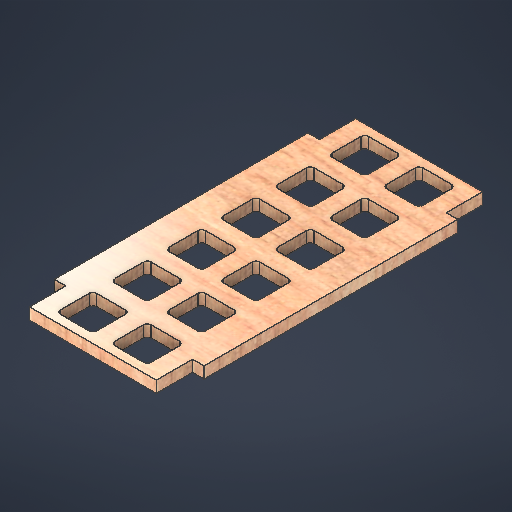
# Autodesk Inventor part: Base-Skiba
Saved by Autodesk Inventor 2027.1 (Build 311270010, 270A)
## iProperties
Created: 2025-11-09
Part Number: Base-Skiba
Material: Generic
Document SubType Name: Modeling
Designer: Nick
Density: 1 g/cm^3
Appearance: Birch - Natural Polished
Mass: 61.0819 g
Surface Area: 284.091 cm^2
Volume: 61.0819 cm^3
Author: Nick
Autodesk Inventor part; units mm, degrees
ref_plane "YZ Plane" through (0, 0, 0) normal (1, 0, 0) x (0, 1, 0)
ref_plane "XZ Plane" through (0, 0, 0) normal (0, 1, 0) x (-1, 0, 0)
ref_plane "XY Plane" through (0, 0, 0) normal (0, 0, 1) x (1, 0, 0)
sketch "Sketch1" plane through (0, 0, 0) normal (0, 1, 0) x (-1, 0, 0)
  line L0 (0, 0) -> (70, 0)
  line L1 (70, 0) -> (70, -180)
  line L2 (70, -180) -> (0, -180)
  line L3 (0, -180) -> (0, 0)
  line L4 (0, 0) -> (4.5, 0)
  line L5 (4.5, 0) -> (4.5, -10) construction
  line L6 (4.5, -10) -> (0, -10) construction
  line L7 (0, -10) -> (0, 0)
  line L8 (4.5, -10) -> (10.85, -10)
  line L9 (10.85, -10) -> (10.85, -30)
  line L10 (10.85, -30) -> (4.5, -30)
  line L11 (4.5, -30) -> (4.5, -10)
  line L12 (4.5, -80) -> (10.85, -80)
  line L13 (10.85, -80) -> (10.85, -100)
  line L14 (10.85, -100) -> (4.5, -100)
  line L15 (4.5, -100) -> (4.5, -80)
  line L16 (4.5, -150) -> (10.85, -150)
  line L17 (10.85, -150) -> (10.85, -170)
  line L18 (10.85, -170) -> (4.5, -170)
  line L19 (4.5, -170) -> (4.5, -150)
  line L20 (35, 0) -> (35, -180) construction
  line L21 (0, -20) -> (-6.35, -20)
  line L22 (-6.35, -20) -> (-6.35, -160)
  line L23 (-6.35, -160) -> (0, -160)
  line L24 (0, -160) -> (0, -20)
  line L25 (65.5, -170) -> (65.5, -150)
  line L26 (70, -20) -> (76.35, -20)
  line L27 (76.35, -20) -> (76.35, -160)
  line L28 (76.35, -160) -> (70, -160)
  line L29 (70, -160) -> (70, -20)
  point P0 (70, -160)
  dimension "d0" = 70
  dimension "d1" = 180
  dimension "d2" = 4.5
  dimension "d3" = 10
  dimension "d8" = 70
  dimension "d30" = 6.35
  dimension "d31" = 140
  constraints: 60 end point, 8 parallel, 6 symmetric about line, 4 horizontal, 4 perpendicular, 2 midpoint, 1 point on line, 1 vertical, 16 other
  measures "d0" distance of L1.end L2.end
  measures "d1" distance of L0.end L1.end
  measures "d2" distance of L5.end L6.end
  measures "d3" distance of L4.end L5.end
  measures "d8" distance of L5.end L12.start
  measures "d30" distance of L23.end L22.end
  measures "d31" distance of L22.end L21.end
extrude "Extrusion1" add sketch "Sketch1" along normal blind 6.35 contours L0 L1 L2 L3 | L3 L23 L22 L21 | L26 L27 L28 L1 | L8 L9 L10 L11 | L12 L13 L14 L15 | L16 L17 L18 L19
sketch "Sketch2" plane through (0, 6.35, 0) normal (0, 1, 0) x (1, 0, 0)
  line L0 (-70, 180) -> (-70, 0) construction
  line L1 (-70, 0) -> (-60, 0) construction
  line L2 (-60, 0) -> (-60, 5) construction
  line L3 (-60, 5) -> (-70, 5) construction
  line L4 (-70, 5) -> (-70, 0) construction
  line L5 (-58, 5) -> (-42, 5)
  line L6 (-40, 7) -> (-40, 23)
  line L7 (-42, 25) -> (-58, 25)
  line L8 (-60, 23) -> (-60, 7)
  arc A0 (-58, 25) -> (-60, 23) centre (-58, 23) ccw
  arc A1 (-42, 5) -> (-40, 7) centre (-42, 7) ccw
  arc A2 (-40, 23) -> (-42, 25) centre (-42, 23) ccw
  arc A3 (-60, 7) -> (-58, 5) centre (-58, 7) ccw
  arc A4 (-60, 37) -> (-58, 35) centre (-58, 37) ccw
  arc A5 (-42, 35) -> (-40, 37) centre (-42, 37) ccw
  line L9 (-60, 53) -> (-60, 37)
  line L10 (-42, 55) -> (-58, 55)
  arc A6 (-58, 55) -> (-60, 53) centre (-58, 53) ccw
  arc A7 (-40, 53) -> (-42, 55) centre (-42, 53) ccw
  line L11 (-40, 37) -> (-40, 53)
  line L12 (-58, 35) -> (-42, 35)
  arc A8 (-60, 67) -> (-58, 65) centre (-58, 67) ccw
  arc A9 (-42, 65) -> (-40, 67) centre (-42, 67) ccw
  line L13 (-60, 83) -> (-60, 67)
  line L14 (-42, 85) -> (-58, 85)
  arc A10 (-58, 85) -> (-60, 83) centre (-58, 83) ccw
  arc A11 (-40, 83) -> (-42, 85) centre (-42, 83) ccw
  line L15 (-40, 67) -> (-40, 83)
  line L16 (-58, 65) -> (-42, 65)
  arc A12 (-60, 97) -> (-58, 95) centre (-58, 97) ccw
  arc A13 (-42, 95) -> (-40, 97) centre (-42, 97) ccw
  line L17 (-60, 113) -> (-60, 97)
  line L18 (-42, 115) -> (-58, 115)
  arc A14 (-58, 115) -> (-60, 113) centre (-58, 113) ccw
  arc A15 (-40, 113) -> (-42, 115) centre (-42, 113) ccw
  line L19 (-40, 97) -> (-40, 113)
  line L20 (-58, 95) -> (-42, 95)
  arc A16 (-30, 7) -> (-28, 5) centre (-28, 7) ccw
  arc A17 (-12, 5) -> (-10, 7) centre (-12, 7) ccw
  line L21 (-30, 23) -> (-30, 7)
  line L22 (-12, 25) -> (-28, 25)
  arc A18 (-28, 25) -> (-30, 23) centre (-28, 23) ccw
  arc A19 (-10, 23) -> (-12, 25) centre (-12, 23) ccw
  line L23 (-10, 7) -> (-10, 23)
  line L24 (-28, 5) -> (-12, 5)
  arc A20 (-30, 37) -> (-28, 35) centre (-28, 37) ccw
  arc A21 (-12, 35) -> (-10, 37) centre (-12, 37) ccw
  line L25 (-30, 53) -> (-30, 37)
  line L26 (-12, 55) -> (-28, 55)
  arc A22 (-28, 55) -> (-30, 53) centre (-28, 53) ccw
  arc A23 (-10, 53) -> (-12, 55) centre (-12, 53) ccw
  line L27 (-10, 37) -> (-10, 53)
  line L28 (-28, 35) -> (-12, 35)
  arc A24 (-30, 67) -> (-28, 65) centre (-28, 67) ccw
  arc A25 (-12, 65) -> (-10, 67) centre (-12, 67) ccw
  line L29 (-30, 83) -> (-30, 67)
  line L30 (-12, 85) -> (-28, 85)
  arc A26 (-28, 85) -> (-30, 83) centre (-28, 83) ccw
  arc A27 (-10, 83) -> (-12, 85) centre (-12, 83) ccw
  line L31 (-10, 67) -> (-10, 83)
  line L32 (-28, 65) -> (-12, 65)
  arc A28 (-30, 97) -> (-28, 95) centre (-28, 97) ccw
  arc A29 (-12, 95) -> (-10, 97) centre (-12, 97) ccw
  line L33 (-30, 113) -> (-30, 97)
  line L34 (-12, 115) -> (-28, 115)
  arc A30 (-28, 115) -> (-30, 113) centre (-28, 113) ccw
  arc A31 (-10, 113) -> (-12, 115) centre (-12, 113) ccw
  line L35 (-10, 97) -> (-10, 113)
  line L36 (-28, 95) -> (-12, 95)
  arc A32 (-60, 127) -> (-58, 125) centre (-58, 127) ccw
  arc A33 (-42, 125) -> (-40, 127) centre (-42, 127) ccw
  line L37 (-60, 143) -> (-60, 127)
  line L38 (-42, 145) -> (-58, 145)
  arc A34 (-58, 145) -> (-60, 143) centre (-58, 143) ccw
  arc A35 (-40, 143) -> (-42, 145) centre (-42, 143) ccw
  line L39 (-40, 127) -> (-40, 143)
  line L40 (-58, 125) -> (-42, 125)
  arc A36 (-30, 127) -> (-28, 125) centre (-28, 127) ccw
  arc A37 (-12, 125) -> (-10, 127) centre (-12, 127) ccw
  line L41 (-30, 143) -> (-30, 127)
  line L42 (-12, 145) -> (-28, 145)
  arc A38 (-28, 145) -> (-30, 143) centre (-28, 143) ccw
  arc A39 (-10, 143) -> (-12, 145) centre (-12, 143) ccw
  line L43 (-10, 127) -> (-10, 143)
  line L44 (-28, 125) -> (-12, 125)
  arc A40 (-60, 157) -> (-58, 155) centre (-58, 157) ccw
  arc A41 (-42, 155) -> (-40, 157) centre (-42, 157) ccw
  line L45 (-60, 173) -> (-60, 157)
  line L46 (-42, 175) -> (-58, 175)
  arc A42 (-58, 175) -> (-60, 173) centre (-58, 173) ccw
  arc A43 (-40, 173) -> (-42, 175) centre (-42, 173) ccw
  line L47 (-40, 157) -> (-40, 173)
  line L48 (-58, 155) -> (-42, 155)
  arc A44 (-30, 157) -> (-28, 155) centre (-28, 157) ccw
  arc A45 (-12, 155) -> (-10, 157) centre (-12, 157) ccw
  line L49 (-30, 173) -> (-30, 157)
  line L50 (-12, 175) -> (-28, 175)
  arc A46 (-28, 175) -> (-30, 173) centre (-28, 173) ccw
  arc A47 (-10, 173) -> (-12, 175) centre (-12, 173) ccw
  line L51 (-10, 157) -> (-10, 173)
  line L52 (-28, 155) -> (-12, 155)
  point P0 (0, 0)
  point P1 (-40, 25)
  point P2 (-40, 5)
  point P3 (-60, 25)
  point P4 (-40, 35)
  point P5 (-60, 55)
  point P6 (-60, 35)
  point P7 (-40, 55)
  point P8 (-40, 65)
  point P9 (-60, 85)
  point P10 (-60, 65)
  point P11 (-40, 85)
  point P12 (-40, 95)
  point P13 (-60, 115)
  point P14 (-60, 95)
  point P15 (-40, 115)
  point P16 (-10, 5)
  point P17 (-30, 25)
  point P18 (-30, 5)
  point P19 (-10, 25)
  point P20 (-10, 35)
  point P21 (-30, 55)
  point P22 (-30, 35)
  point P23 (-10, 55)
  point P24 (-10, 65)
  point P25 (-30, 85)
  point P26 (-30, 65)
  point P27 (-10, 85)
  point P28 (-10, 95)
  point P29 (-30, 115)
  point P30 (-30, 95)
  point P31 (-10, 115)
  point P32 (-40, 125)
  point P33 (-60, 145)
  point P34 (-60, 125)
  point P35 (-40, 145)
  point P36 (-10, 125)
  point P37 (-30, 145)
  point P38 (-30, 125)
  point P39 (-10, 145)
  point P40 (-40, 155)
  point P41 (-60, 175)
  point P42 (-60, 155)
  point P43 (-40, 175)
  point P44 (-10, 155)
  point P45 (-30, 175)
  point P46 (-30, 155)
  point P47 (-10, 175)
  dimension "d15" = 10
  dimension "d16" = 5
  dimension "d17" = 20
  dimension "d18" = 20
  dimension "d19" = 2
  dimension "d22" = 30
  dimension "d25" = 30
  constraints: 104 end point, 96 point on circle, 96 point on line, 48 centre point, 8 tangent, 4 parallel, 3 equal radius, 3 horizontal, 2 perpendicular, 1 vertical, 264 other
  measures "d15" distance of L3.end L2.end
  measures "d16" distance of L2.end L1.end
  measures "d17" distance of point (-60, 25) point (-40, 25)
  measures "d18" distance of point (-40, 25) point (-40, 5)
  measures "d19" radius of A0
  measures "d22" distance of L8.end L9.end
  measures "d25" distance of L8.end L21.end
extrude "Extrusion2" cut sketch "Sketch2" against normal blind 6.35
body "Solid1"
